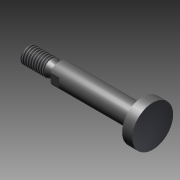
# Autodesk Inventor part: 536233 ADN-15-P-A_(KS)
Saved by Autodesk Inventor 2011 SP1 (Build 150282100, 282)
## iProperties
Created: 2018-05-29
Part Number: 536233 ADN-15-P-A_(KS)
Catalog Web Link: www.cadenas.de
Description: ADN-(KS)-Compact cylinder - piston rod
Vendor: FESTO
Document SubType Name: Modeling
Designer: psAdmin
Manufacturer: FESTO
Mass: 5.48187 g
Surface Area: 26.0559 cm^2
Volume: 5.48187 cm^3
Density: 1 g/cm^3
Category: PARTsolutions
Company: FESTO
Title: 536233 ADN-15-P-A_(KS)
Author: Cadenas PARTsolutions
Comments: Compact cylinder - piston rod
PSOL_IDENT_0: {$CADENAS_DATA\23d-libs\festo\parts\a\adn\parts\adn_ks.prj},229 {VTYP=3D},{NB=536233 ADN-15-P-A_(KS)
PSOL_IDENT_1: },{LINA=536233 ADN-15-P-A_(KS)},{NN=ADN-(KS)},{DATE=06.10.2015 11:54:02},{GEOMDATE=23.09.2015 12:10:
PSOL_IDENT_2: 00},{VERSION=},{LINEID=8190},{LINESUBID=-1},{WBVAR=DF,HUB,TH,Q,S2S20,K2,K5,K8,K10,S1,TT,R8}  {NB=536
PSOL_IDENT_3: 233 ADN-15-P-A_(KS)},{LINA=536233 ADN-15-P-A_(KS)},{KT=536233},{TNR=536233},{AUSF=ADN},{DF=P},{GA=A}
PSOL_IDENT_4: ,{WHX=5.5},{WH0=5.500},{WH1=0.000},{WH2=10.500},{WH3=5.500},{WHX1=5.5},{WHX2=6.25},{WH=5.5},{ZM=49.5
PSOL_IDENT_5: 00},{ZM2=49.500},{ZB=42.500},{ZB1=0.000},{ZB2=42.500},{ZB6=47.500},{ZA=37.000},{KDM=20},{HUBP=-},{HU
PSOL_IDENT_6: B=15},{HUB1=[1-300]},{HUB2=[1-200]},{HUB3=0},{HUB4=[1-300]},{TH=A},{THC='A','I'},{Q=-},{VAR1C='-','Q'
PSOL_IDENT_7: },{S2S20=-},{VAR2C='-','S2','S20'},{VAR22C='-','S2'},{VAR222C='-','S2','S20'},{K2=0},{VAR3C=0,[1-20]
PSOL_IDENT_8: },{VAR33C=0,[1-20]},{K5=-},{K5A='-','M10','M10X1,25'},{K5I='-','M5'},{K5S1A='-'},{K5S1I='-'},{K5C='-'
PSOL_IDENT_9: ,'M10','M10X1,25'},{K5N=0},{K5P=0},{K5T=},{K8=0},{K10=-},{K10A='-','K10'},{K10N=},{S1=-},{TT=-},{TT1='
PSOL_IDENT_10: -','TT'},{R8=-},{R81='-','R8'},{VAR4C=0,[1-300]},{VAR5C='-','S6'},{VAR6C='-'},{VAR66C='-'},{VAR7C='-'
PSOL_IDENT_11: ,'R3'},{HUBALG=[1-300]},{A=16.000},{A1=0.000},{AF=14.000},{AF1=0.000},{AF2=12.000},{AF3=0.000},{AF5=
PSOL_IDENT_12: 12.000},{AF7=0.000},{D8=3.800},{D9=6.000},{KF=M6},{KFN=6.000},{KF1=-},{KF1C=0.0000},{KF2=-},{KF2C=0.
PSOL_IDENT_13: 0000},{KF3=M5},{KF3C=5.0000},{KF5=M5},{KF5N=5},{KF7=-},{KF7N=0},{KK=M8},{KKN=8},{KKP=1.25},{KK1=-},{
PSOL_IDENT_14: KK1N=0.0000},{KK1P=0.00},{L2=37.000},{L8=2.000},{MM=10.000},{MM1=0.000},{PL=6.000},{SF=9},{SF1=0},{S
PSOL_IDENT_15: F3=9.0},{WL=4.200},{WL1=0.000},{QN=},{S2N=},{S1N=},{K2N=},{K8N=},{KKC3=6.200},{KKF2=0.600},{KKD5=1.5
PSOL_IDENT_16: 00},{KKE2=20.000},{K5C3=0},{K5F2=0},{K5D5=0},{KK1C3=0.000},{KK1F2=0.000},{KK1D5=0.000},{KK1E2=0.000}
PSOL_IDENT_17: ,{L100S1=0.000},{L101S1=0.000},{L102S1=0.000},{L103S1=0.000},{D100S1=0.000},{L100=0.400},{L101=2.600
PSOL_IDENT_18: },{L102=14.000},{L103=18.000},{D100=6.400},{L100Q=0.400},{L101Q=2.600},{L101K5=2.000},{L102Q=12.000}
PSOL_IDENT_19: ,{L103Q=15.500},{D100Q=5.300},{L100S1K5=0.000},{L101S1K5=0.000},{L102S1K5=0.000},{L103S1K5=0.000},{D
PSOL_IDENT_20: 100S1K5=0.000},{VERS=1},{TTN=},{R8N=},{D20=0.000},{XF31=4.000},{B31=4.000},{DFALG='P','PPS'}
NN: ADN-(KS)
NT: Compact cylinder - piston rod
NB: 536233 ADN-15-P-A_(KS)
NBSYN: $TNR. $AUSF.-$HUB.-$DF.-$TH.$QN.$S2N.$K2N.$K5T.$K8N.$K10N.$S1N.$TTN.$R8N._(KS)
LINA: 536233 ADN-15-P-A_(KS)
TNR: 536233
AUSF: ADN
DF: P
GA: A
WHX: 5.500
WH0: 5.500
WH1: 0.000
WH2: 10.500
WH3: 5.500
WHX1: 5.500
WHX2: 6.250
WH: 5.500
ZM: 49.500
ZM2: 49.500
ZB: 42.500
ZB1: 0.000
ZB2: 42.500
ZB6: 47.500
ZA: 37.000
KDM: 20
HUBP: -
HUB: 15
TH: A
Q: -
S2S20: -
K2: 0
K5: -
K8: 0
K10: -
S1: -
TT: -
R8: -
A: 16.000
A1: 0.000
AF: 14.000
AF1: 0.000
AF2: 12.000
AF3: 0.000
AF5: 12.000
AF7: 0.000
D8: 3.800
D9: 6.000
KF: M6
KF1: -
KF2: -
KF3: M5
KF5: M5
KF7: -
KK: M8
KK1: -
L2: 37.000
L8: 2.000
MM: 10.000
MM1: 0.000
PL: 6.000
SF: 9
SF1: 0
SF3: 9.0
WL: 4.200
WL1: 0.000
L101K5: 2.000
D20: 0.000
XF31: 4.000
B31: 4.000
SUPPLIER: FESTO
ARTICLENO: 536233 ADN-15-P-A_(KS)
BOMINFO: 536233 ADN-15-P-A_(KS)
CREATOR: CADENAS GmbH
Autodesk Inventor part; units mm, degrees
ref_plane "YZ Plane" through (0, 0, 0) normal (1, 0, 0) x (0, 1, 0)
ref_plane "XZ Plane" through (0, 0, 0) normal (0, 1, 0) x (-1, 0, 0)
ref_plane "XY Plane" through (0, 0, 0) normal (0, 0, 1) x (1, 0, 0)
sketch "Sketch_1" plane through (0, 0, 0) normal (0, 0, 1) x (1, 0, 0)
  line L0 (40, 0) -> (-5.5, 0)
  line L1 (-5.5, 0) -> (-5.5, 5)
  line L2 (-5.5, 5) -> (40, 5)
  line L3 (40, 5) -> (40, 0)
  line L4 (40, 0) -> (-5.5, 0)
  constraints: 10 end point
revolve "Revolution1" add sketch "Sketch_1" angle 360 about axis through (40, 0, 0) along (1, 0, 0)
sketch "Sketch_11" plane through (0, 0, 0) normal (0, 0, 1) x (1, 0, 0)
  line L0 (40, 0) -> (35, 0)
  line L1 (35, 0) -> (35, 10)
  line L2 (35, 10) -> (40, 10)
  line L3 (40, 10) -> (40, 0)
  line L4 (40, 0) -> (35, 0)
  constraints: 10 end point
revolve "Revolution2" add sketch "Sketch_11" angle 360 about axis through (40, 0, 0) along (1, 0, 0)
sketch "Sketch_19" plane through (0, 0, 0) normal (0, 0, 1) x (1, 0, 0)
  line L0 (-4.5, 0) -> (-21.5, 0)
  line L1 (-21.5, 0) -> (-21.5, 3.233)
  line L2 (-21.5, 3.233) -> (-20.733, 4)
  line L3 (-20.733, 4) -> (-9.4727, 4)
  line L4 (-9.4727, 4) -> (-7.0994, 3.1362)
  arc A0 (-7.0994, 3.1362) -> (-6.8942, 3.1) centre (-6.8942, 3.7) ccw
  line L5 (-6.8942, 3.1) -> (-6.1, 3.1)
  arc A1 (-6.1, 3.1) -> (-5.5, 3.7) centre (-6.1, 3.7) ccw
  line L6 (-5.5, 3.7) -> (-5.5, 4)
  line L7 (-5.5, 4) -> (-4.5, 4)
  line L8 (-4.5, 4) -> (-4.5, 0)
  line L9 (-4.5, 0) -> (-21.5, 0)
  constraints: 20 end point, 4 point on circle, 2 centre point
revolve "Revolution3" add sketch "Sketch_19" angle 360 about axis through (-4.5, 0, 0) along (1, 0, 0)
thread "Thread1" size "M8x1.25" class "6g" standard "ISO Metric profile" full length
sketch "Sketch_20" plane through (0, 0, 0) normal (0, 0, 1) x (1, 0, 0)
  line L0 (-32, -14.5) -> (4.4735, -14.5)
  line L1 (4.4735, -14.5) -> (-1.3, -4.5)
  line L2 (-1.3, -4.5) -> (-5.5, -4.5)
  line L3 (-5.5, -4.5) -> (-5.5, -9.5)
  line L4 (-5.5, -9.5) -> (-26.5, -9.5)
  line L5 (-26.5, -9.5) -> (-26.5, 9.5)
  line L6 (-26.5, 9.5) -> (-5.5, 9.5)
  line L7 (-5.5, 9.5) -> (-5.5, 4.5)
  line L8 (-5.5, 4.5) -> (-1.3, 4.5)
  line L9 (-1.3, 4.5) -> (4.4735, 14.5)
  line L10 (4.4735, 14.5) -> (-32, 14.5)
  line L11 (-32, 14.5) -> (-32, -14.5)
  constraints: 24 end point
extrude "Extrusion1" cut sketch "Sketch_20" along normal mid plane 20
ref_plane "FDT_PIRODACC_M1_XY" through (-13.5, 0, 0) normal (-1, 0, 0) x (0, 1, 0)
ref_plane "FDT_PIRODACC_M1_YZ" through (-13.5, 0, 0) normal (0, 1, 0) x (0, 0, -1)
ref_plane "FDT_PIRODACC_M1_ZX" through (-13.5, 0, 0) normal (0, 0, -1) x (-1, 0, 0)
ref_plane "NUT1_XY" through (-11.5, 0, 0) normal (1, 0, 0) x (0, 0, -1)
ref_plane "NUT1_YZ" through (-11.5, 0, 0) normal (0, 0, -1) x (0, 1, 0)
ref_plane "NUT1_ZX" through (-11.5, 0, 0) normal (0, 1, 0) x (1, 0, 0)
ref_plane "PISTON_XY" through (40, 0, 0) normal (1, 0, 0) x (0, 0, -1)
ref_plane "PISTON_YZ" through (40, 0, 0) normal (0, 0, -1) x (0, 1, 0)
ref_plane "PISTON_ZX" through (40, 0, 0) normal (0, 1, 0) x (1, 0, 0)
body "Solid1"
